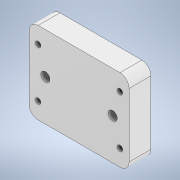
# Autodesk Inventor part: ImpresionSoporte
Saved by Autodesk Inventor 2021 (Build 250183000, 183)
## iProperties
Created: 2022-06-04
Part Number: ImpresionSoporte
Material: Plástico ABS
Document SubType Name: Modeling
Designer: 79449
Density: 1.06 g/cm^3
Appearance: Suave - Blanco
Author: 79449
Autodesk Inventor part; units mm, degrees
ref_plane "YZ Plane" through (0, 0, 0) normal (1, 0, 0) x (0, 1, 0)
ref_plane "XZ Plane" through (0, 0, 0) normal (0, 1, 0) x (-1, 0, 0)
ref_plane "XY Plane" through (0, 0, 0) normal (0, 0, 1) x (1, 0, 0)
sketch "Boceto1" plane through (0, 0, 0) normal (0, 0, 1) x (1, 0, 0)
  circle A0 centre (-22.5, 13.5) radius 1.5
  circle A1 centre (22.5, 13.5) radius 1.5
  line L0 (-22.5, 13.5) -> (22.5, 13.5) construction
  line L1 (-22.5, 13.5) -> (22.5, 13.5) construction
  line L2 (0, 13.5) -> (0, 0) construction
  line L3 (27.5, -22.5) -> (-27.5, -22.5)
  line L4 (-27.5, -22.5) -> (-27.5, 22.5)
  line L5 (-27.5, 22.5) -> (27.5, 22.5)
  line L6 (27.5, 22.5) -> (27.5, -22.5)
  line L7 (27.5, -22.5) -> (-27.5, 22.5) construction
  line L8 (-27.5, -22.5) -> (27.5, 22.5) construction
  line L9 (-27.5, 0) -> (27.5, 0) construction
  circle A2 centre (-22.5, -13.5) radius 1.5
  circle A3 centre (22.5, -13.5) radius 1.5
  circle A4 centre (18.5, 0) radius 2.5
  circle A5 centre (-18.5, 0) radius 2.5
  dimension "d2" = 3
  dimension "d3" = 3
  dimension "d10" = 45
  dimension "d11" = 55
  dimension "d12" = 45
  dimension "d15" = 13.5
  dimension "d17" = 18.5
  dimension "d18" = 5
  constraints: 20 end point, 6 centre point, 5 midpoint, 3 equal length, 3 symmetric about line, 2 horizontal, 1 perpendicular, 1 point on line, 1 vertical, 3 other
  measures "d2" diameter of A0
  measures "d3" diameter of A1
  measures "d10" distance of L0.end L0.start
  measures "d11" distance of L3.start L3.end
  measures "d12" distance of L5.end L3.start
  measures "d15" distance from line of L2.end L0
  measures "d17" distance of A4.centre L2.end
  measures "d18" diameter of A4
extrude "Extrusión1" add sketch "Boceto1" along normal blind 12
fillet "Empalme1" radius 5 4 edges at (27.5, 22.5, 6) (27.5, -22.5, 6) (-27.5, -22.5, 6) (-27.5, 22.5, 6)
